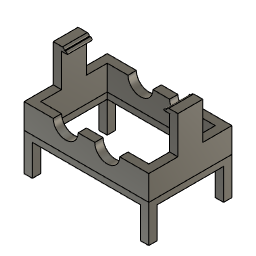
3D Shredder Machine (Autodesk Fusion 360 design; units mm, degrees)
Autodesk Fusion 360 part; units mm, degrees
sketch "base_pillars" plane through (0, 0, 0) normal (0, 0, 1) x (1, 0, 0) in component "Base"
  line L0 (75, 50) -> (-75, 50)
  line L1 (-75, 50) -> (-75, -50)
  line L2 (-75, -50) -> (75, -50)
  line L3 (75, -50) -> (75, 50)
  line L4 (75, 50) -> (-75, -50) construction
  line L5 (-75, 50) -> (75, -50) construction
  line L6 (-75, -50) -> (-65, -50)
  line L7 (-65, -50) -> (-65, -40)
  line L8 (-65, -40) -> (-75, -40)
  line L9 (-75, -40) -> (-75, -50)
  line L10 (-75, 50) -> (-65, 50)
  line L11 (-65, 50) -> (-65, 40)
  line L12 (-65, 40) -> (-75, 40)
  line L13 (-75, 40) -> (-75, 50)
  line L14 (75, 50) -> (65, 50)
  line L15 (65, 50) -> (65, 40)
  line L16 (65, 40) -> (75, 40)
  line L17 (75, 40) -> (75, 50)
  line L18 (75, -50) -> (65, -50)
  line L19 (65, -50) -> (65, -40)
  line L20 (65, -40) -> (75, -40)
  line L21 (75, -40) -> (75, -50)
  dimension "d1" = 150
  dimension "d2" = 100
  dimension "d3" = 10
  dimension "d4" = 10
  dimension "d5" = 10
  dimension "d6" = 10
  dimension "d7" = 10
  dimension "d8" = 10
  dimension "d9" = 10
  dimension "d10" = 10
  constraint horizontal L0
  constraint perpendicular L0 L1
  constraint parallel L0 L2
  constraint parallel L1 L3
  constraint coincident L4 origin
  constraint coincident L5 origin
  constraint horizontal L6
  constraint vertical L7
  constraint horizontal L8
  constraint vertical L9
  constraint horizontal L10
  constraint vertical L11
  constraint horizontal L12
  constraint vertical L13
  constraint horizontal L14
  constraint vertical L15
  constraint horizontal L16
  constraint vertical L17
  constraint horizontal L18
  constraint vertical L19
  constraint horizontal L20
  constraint vertical L21
  measures "d1" distance of L1.end L2.end
  measures "d2" distance of L0.end L1.end
  measures "d3" distance of L1.end L6.end
  measures "d4" distance of L1.end L8.end
  measures "d5" distance of L0.end L10.end
  measures "d6" distance of L0.end L12.end
  measures "d7" distance of L0.start L14.end
  measures "d8" distance of L0.start L16.end
  measures "d9" distance of L2.end L18.end
  measures "d10" distance of L2.end L20.end
extrude "Extrude1" add sketch "base_pillars" along normal blind 45 contours L0 L3 L14 L15 L16 L17 | L0 L1 L10 L11 L12 L13 | L2 L3 L18 L19 L20 L21 | L1 L2 L6 L7 L8 L9 makes body 1 at (-65, 46.6667, 15) makes body 2 at (75, 43.3333, 15) makes body 3 at (-68.3333, -40, 15) makes body 4 at (75, -46.6667, 15) in component "Base"
sketch "base_side_1" plane through (0, 40, 0) normal (0, -1, 0) x (1, 0, 0) in component "Base"
  line L0 (-75, 0) -> (-65, 0)
  line L1 (-65, 0) -> (-65, 45)
  line L2 (-65, 45) -> (-75, 45)
  line L3 (-75, 45) -> (-75, 0)
  line L4 (-75, 45) -> (-65, 45)
  line L5 (-65, 45) -> (-65, 37.5)
  line L6 (-65, 37.5) -> (-75, 37.5)
  line L7 (-75, 37.5) -> (-75, 45)
  dimension "d13" = 10
  dimension "d14" = 7.5
  constraint horizontal L4
  constraint vertical L5
  constraint horizontal L6
  constraint vertical L7
  constraint coincident L2.end L3.start
  measures "d13" distance of L2.end L1.end
  measures "d14" distance of L2.end L6.end
extrude "Extrude2" add sketch "base_side_1" along normal blind 80 contours L1 L2 L3 L4 L5 L6 L7 bodies 1 3 in component "Base"
sketch "base_side_2_and_3" plane through (-65, 0, 0) normal (1, 0, 0) x (0, 1, 0) in component "Base"
  line L0 (40, 0) -> (50, 0)
  line L1 (50, 0) -> (50, 45)
  line L2 (50, 45) -> (-50, 45)
  line L3 (-50, 45) -> (-50, 0)
  line L4 (-50, 0) -> (-40, 0)
  line L5 (-40, 0) -> (-40, 37.5)
  line L6 (-40, 37.5) -> (40, 37.5)
  line L7 (40, 37.5) -> (40, 0)
  line L8 (-50, 45) -> (-40, 45)
  line L9 (-40, 45) -> (-40, 37.5)
  line L10 (-40, 37.5) -> (-50, 37.5)
  line L11 (-50, 37.5) -> (-50, 45)
  line L12 (40, 37.5) -> (50, 37.5)
  line L13 (50, 37.5) -> (50, 45)
  line L14 (50, 45) -> (40, 45)
  line L15 (40, 45) -> (40, 37.5)
  constraint horizontal L8
  constraint vertical L9
  constraint horizontal L10
  constraint vertical L11
  constraint coincident L5.end L6.start
  constraint coincident L2.end L3.start
  constraint horizontal L12
  constraint vertical L13
  constraint horizontal L14
  constraint vertical L15
  constraint coincident L1.end L2.start
  constraint coincident L6.end L7.start
extrude "Extrude3" add sketch "base_side_2_and_3" along normal blind 130 contours L1 L2 L12 L13 L14 L15 | L2 L3 L8 L9 L10 L11 bodies 1 2 4 in component "Base"
sketch "base_side_4" plane through (0, -40, 0) normal (0, 1, 0) x (-1, 0, 0) in component "Base"
  line L0 (-75, 0) -> (-65, 0)
  line L1 (-65, 0) -> (-65, 37.5)
  line L2 (-65, 37.5) -> (65, 37.5)
  line L3 (65, 37.5) -> (65, 45)
  line L4 (65, 45) -> (-75, 45)
  line L5 (-75, 45) -> (-75, 0)
  line L6 (-75, 45) -> (-65, 45)
  line L7 (-65, 45) -> (-65, 37.5)
  line L8 (-65, 37.5) -> (-75, 37.5)
  line L9 (-75, 37.5) -> (-75, 45)
  constraint horizontal L6
  constraint vertical L7
  constraint horizontal L8
  constraint vertical L9
  constraint coincident L1.end L2.start
  constraint coincident L4.end L5.start
extrude "Extrude4" add sketch "base_side_4" along normal blind 80 contours L4 L5 L6 L7 L8 L9 bodies 1 in component "Base"
sketch "walls" plane through (0, 0, 45) normal (0, 0, 1) x (-1, 0, 0) in component "Lower container"
  line L0 (-75, 50) -> (-75, -50)
  line L1 (-75, -50) -> (75, -50)
  line L2 (75, -50) -> (75, 50)
  line L3 (75, 50) -> (-75, 50)
  line L4 (-65, -40) -> (-65, 40)
  line L5 (-65, 40) -> (65, 40)
  line L6 (65, 40) -> (65, -40)
  line L7 (65, -40) -> (-65, -40)
  line L8 (75, 50) -> (-75, 50)
  line L9 (-75, 50) -> (-75, 40)
  line L10 (-75, 40) -> (75, 40)
  line L11 (75, 40) -> (75, 50)
  line L12 (-75, 40) -> (-65, 40)
  line L13 (-65, 40) -> (-65, -50)
  line L14 (-65, -50) -> (-75, -50)
  line L15 (-75, -50) -> (-75, 40)
  line L16 (-65, -50) -> (75, -50)
  line L17 (75, -50) -> (75, -40)
  line L18 (75, -40) -> (-65, -40)
  line L19 (-65, -40) -> (-65, -50)
  line L20 (75, -40) -> (65, -40)
  line L21 (65, -40) -> (65, 40)
  line L22 (65, 40) -> (75, 40)
  line L23 (75, 40) -> (75, -40)
  line L24 (65, 40) -> (75, 40)
  line L25 (75, 40) -> (75, 50)
  line L26 (75, 50) -> (65, 50)
  line L27 (65, 50) -> (65, 40)
  line L28 (-75, 40) -> (-65, 40)
  line L29 (-65, 40) -> (-65, 50)
  line L30 (-65, 50) -> (-75, 50)
  line L31 (-75, 50) -> (-75, 40)
  line L32 (65, -40) -> (75, -40)
  line L33 (75, -40) -> (75, -50)
  line L34 (75, -50) -> (65, -50)
  line L35 (65, -50) -> (65, -40)
  line L36 (-65, -40) -> (-75, -40)
  line L37 (-75, -40) -> (-75, -50)
  line L38 (-75, -50) -> (-65, -50)
  line L39 (-65, -50) -> (-65, -40)
  constraint horizontal L8
  constraint vertical L9
  constraint horizontal L10
  constraint vertical L11
  constraint coincident L0 L9.end
  constraint coincident L2.end L3.start
  constraint horizontal L12
  constraint vertical L13
  constraint horizontal L14
  constraint vertical L15
  constraint coincident L1 L13.end
  constraint horizontal L16
  constraint vertical L17
  constraint horizontal L18
  constraint vertical L19
  constraint coincident L2 L17.end
  constraint horizontal L20
  constraint vertical L21
  constraint horizontal L22
  constraint vertical L23
  constraint coincident L5.end L6.start
  constraint horizontal L24
  constraint vertical L25
  constraint horizontal L26
  constraint vertical L27
  constraint horizontal L28
  constraint vertical L29
  constraint horizontal L30
  constraint vertical L31
  constraint coincident L8 L29.end
  constraint horizontal L32
  constraint vertical L33
  constraint horizontal L34
  constraint vertical L35
  constraint coincident L1.end L2.start
  constraint coincident L6.end L7.start
  constraint horizontal L36
  constraint vertical L37
  constraint horizontal L38
  constraint vertical L39
  constraint coincident L0.end L1.start
  constraint coincident L4.start L7.end
extrude "Extrude1'" add sketch "walls" along normal blind 30 separate body contours L0 L3 L8 L9 L10 L12 L28 L29 L30 L31 | L3 L5 L8 L10 L27 L29 | L0 L1 L13 L14 L15 L19 L36 L37 L38 L39 | L2 L3 L8 L10 L11 L22 L24 L25 L26 L27 | L1 L7 L13 L16 L18 L19 L35 L39 | L1 L2 L16 L17 L18 L20 L32 L33 L34 L35 makes body 5 at (-25, 40, 55) makes body 6 at (-25, -50, 55) in component "Lower container"
sketch "holes" plane through (0, 50, 0) normal (0, 1, 0) x (-1, 0, 0) in component "Lower container"
  line L0 (-75, 45) -> (75, 45)
  line L1 (75, 45) -> (75, 75)
  line L2 (75, 75) -> (-75, 75)
  line L3 (-75, 75) -> (-75, 45)
  circle A0 centre (-25, 75) radius 15
  circle A1 centre (25, 75) radius 15
  dimension "d25" = 30
  measures "d25" diameter of A1
extrude "Extrude2'" cut sketch "holes" against normal blind 100 contours L2 A0 | L2 A1 picked at (-26.1126, 70.1254) picked at (23.8874, 70.1254) bodies 5 6 in component "Lower container"
extrude "Extrude3'" add sketch "walls" along normal blind 30 contours L0 L4 L10 L12 L13 L15 L28 L36 | L2 L6 L10 L18 L20 L21 L22 L23 L24 L32 bodies 5 6 in component "Lower container"
sketch "extension_of_wall" plane through (0, 0, 75) normal (0, 0, 1) x (-1, 0, 0) in component "Lower container"
  line L0 (-40, -50) -> (-40, -40)
  line L1 (-40, -40) -> (-65, -40)
  line L2 (-65, -40) -> (-65, 40)
  line L3 (-65, 40) -> (-40, 40)
  line L4 (-40, 40) -> (-40, 50)
  line L5 (-40, 50) -> (-75, 50)
  line L6 (-75, 50) -> (-75, -50)
  line L7 (-75, -50) -> (-40, -50)
  line L8 (-75, 50) -> (-75, 20)
  line L9 (-75, -50) -> (-75, -20)
  line L10 (-75, 20) -> (-75, 15)
  line L11 (-75, -20) -> (-75, -15)
  line L12 (-75, 15) -> (-65, 15)
  line L13 (-65, 15) -> (-65, -15)
  line L14 (-65, -15) -> (-75, -15)
  line L15 (-75, -15) -> (-75, 15)
  dimension "d30" = 30
  dimension "d31" = 30
  dimension "d32" = 5
  dimension "d33" = 5
  constraint coincident L5.end L6.start
  constraint perpendicular L5 L8
  constraint coincident L6.end L7.start
  constraint coincident L6 L9.end
  constraint parallel L6 L10
  constraint parallel L6 L11
  constraint horizontal L12
  constraint vertical L13
  constraint horizontal L14
  constraint vertical L15
  constraint coincident L2 L13.end
  measures "d30" distance of L5.end L8.end
  measures "d31" distance of L6.end L9.end
  measures "d32" distance of L8.end L10.end
  measures "d33" distance of L9.end L11.end
extrude "Extrude4'" add sketch "extension_of_wall" along normal blind 45 separate body contours L2 L6 L12 L13 L14 L15 makes body 7 in component "Lower container"
sketch "blocking_part_for upper_container" plane through (65, 0, 0) normal (-1, 0, 0) x (0, -1, 0) in component "Lower container"
  line L0 (-40, 45) -> (40, 45)
  line L1 (40, 45) -> (40, 75)
  line L2 (40, 75) -> (-40, 75)
  line L3 (-40, 75) -> (-40, 45)
  line L4 (-15, 120) -> (15, 120)
  line L5 (15, 120) -> (15, 117.5)
  line L6 (15, 117.5) -> (-15, 117.5)
  line L7 (-15, 117.5) -> (-15, 120)
  line L8 (-15, 117.5) -> (15, 117.5)
  line L9 (15, 117.5) -> (15, 115)
  line L10 (15, 115) -> (-15, 115)
  line L11 (-15, 115) -> (-15, 117.5)
  dimension "d36" = 2.5
  dimension "d37" = 2.5
  constraint horizontal L4
  constraint vertical L5
  constraint horizontal L6
  constraint vertical L7
  constraint horizontal L8
  constraint vertical L9
  constraint horizontal L10
  constraint vertical L11
  measures "d36" distance of L4.start L6.end
  measures "d37" distance of L6.end L10.end
extrude "Extrude5" add sketch "blocking_part_for upper_container" along normal blind 3.5 contours L4 L5 L6 L7 L8 bodies 5 7 in component "Lower container"
extrude "Extrude6" add sketch "blocking_part_for upper_container" along normal blind 7 contours L6 L8 L9 L10 L11 bodies 7 5 in component "Lower container"
copy_body "CopyPasteBodies1" bodies 7 makes body 8 in component "Lower container"
move_body "Move1" bodies 8 to x (-1, 0, 0) y (0, -1, 0) z (0, 0, 1) at (0, 0, 0) in component "Lower container"
combine "Combine1" operation add target body 7 tool bodies 5 in component "Lower container"
combine "Combine2" operation add target body 7 tool bodies 8 in component "Lower container"
fillet "Fillet1" radius 2.5 1 edges at (-58, 0, 117.5) on bodies 7 in component "Lower container"
fillet "Fillet2" radius 2.5 1 edges at (-61.5, 0, 120) on bodies 7 in component "Lower container"
fillet "Fillet3" radius 2.5 2 edges at (61.5, 0, 120) (58, 0, 117.5) on bodies 7 in component "Lower container"
component "Base" placed x (1, 0, 0) y (0, 1, 0) z (0, 0, 1) at (0, 0, 0)
component "Lower container" placed x (1, 0, 0) y (0, 1, 0) z (0, 0, 1) at (0, 0, 0)
component "Shredder" placed x (1, 0, 0) y (0, 1, 0) z (0, 0, 1) at (0, 0, 0)
component "Upper container" placed x (1, 0, 0) y (0, 1, 0) z (0, 0, 1) at (0, 0, 0)
component "Crank" placed x (1, 0, 0) y (0, 1, 0) z (0, 0, 1) at (0, 0, 0)
component "Recipient" placed x (1, 0, 0) y (0, 1, 0) z (0, 0, 1) at (0, 0, 0)
named bodies: "base", "lower_container"
